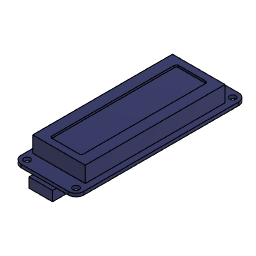
LCD1602 RGB Module v2 (Autodesk Fusion 360 design; units mm, degrees)
Autodesk Fusion 360 part; units mm, degrees
sketch "Skizze1" plane through (0, 0, 0) normal (0, 0, 1) x (1, 0, 0)
  line L0 (4, 0) -> (28, 0)
  line L1 (32, 4) -> (32, 83)
  line L2 (28, 87) -> (4, 87)
  line L3 (0, 83) -> (0, 4)
  circle A0 centre (3.5, 3.5) radius 1.6
  circle A1 centre (28.5, 3.5) radius 1.6
  circle A2 centre (3.5, 83.5) radius 1.6
  circle A3 centre (28.5, 83.5) radius 1.6
  arc A4 (4, 87) -> (0, 83) centre (4, 83) ccw
  arc A5 (32, 83) -> (28, 87) centre (28, 83) ccw
  arc A6 (0, 4) -> (4, 0) centre (4, 4) ccw
  arc A7 (28, 0) -> (32, 4) centre (28, 4) ccw
  point P0 (32, 0)
  point P1 (0, 87)
  dimension "d1" = 32
  dimension "d2" = 87
  dimension "d3" = 3.2
  dimension "d4" = 3.5
  dimension "d5" = 3.5
  dimension "d8" = 25
  dimension "d9" = 80
  dimension "d10" = 4
  constraint horizontal L0
  constraint vertical L1
  constraint horizontal L2
  constraint vertical L3
  constraint coincident P1 L2
  constraint coincident P1 L3
  constraint tangent L2 A4
  constraint tangent L3 A4
  constraint tangent L1 A5
  constraint tangent L2 A5
  constraint equal A4 A5
  constraint coincident origin L0
  constraint coincident origin L3
  constraint tangent L0 A6
  constraint tangent L3 A6
  constraint equal A4 A6
  constraint coincident P0 L0
  constraint coincident P0 L1
  constraint tangent L0 A7
  constraint tangent L1 A7
  constraint equal A4 A7
  measures "d1" distance of origin P0
  measures "d2" distance of origin P1
  measures "d3" diameter of A0
  measures "d4" distance of L0 A0.centre
  measures "d5" distance of L3 A0.centre
  measures "d10" radius of A4
extrude "Extrusion1" add sketch "Skizze1" along normal blind 1.6
sketch "Skizze2" plane through (0, 0, 1.6) normal (0, 0, 1) x (-1, 0, 0)
  circle A0 centre (-28.5, -3.5) radius 1.6
  circle A1 centre (-3.5, -3.5) radius 1.6
  circle A2 centre (-3.5, -83.5) radius 1.6
  circle A3 centre (-28.5, -83.5) radius 1.6
  arc A4 (-28, 0) -> (-32, -4) centre (-28, -4) ccw
  line L0 (-32, -4) -> (-32, -83)
  arc A5 (-32, -83) -> (-28, -87) centre (-28, -83) ccw
  line L1 (-28, -87) -> (-4, -87)
  arc A6 (-4, -87) -> (0, -83) centre (-4, -83) ccw
  line L2 (0, -83) -> (0, -4)
  arc A7 (0, -4) -> (-4, 0) centre (-4, -4) ccw
  line L3 (-4, 0) -> (-28, 0)
  line L4 (-2.08, -7.8) -> (-28.88, -7.8)
  line L5 (-28.88, -7.8) -> (-28.88, -79.1)
  line L6 (-28.88, -79.1) -> (-2.08, -79.1)
  line L7 (-2.08, -79.1) -> (-2.08, -7.8)
  dimension "d13" = 26.8
  dimension "d14" = 71.3
  dimension "d15" = 7.8
  dimension "d16" = 2.08
  constraint horizontal L4
  constraint vertical L5
  constraint horizontal L6
  constraint vertical L7
  measures "d13" distance of L4.start L4.end
  measures "d14" distance of L4.start L6.end
  measures "d15" distance of L3 L4
  measures "d16" distance of L2 L7
extrude "Extrusion2" add sketch "Skizze2" along normal blind 8.1 contours L4 L5 L6 L7
sketch "Skizze3" plane through (0, 0, 9.7) normal (0, 0, 1) x (-1, 0, 0)
  line L0 (-2.08, -79.1) -> (-2.08, -7.8)
  line L1 (-2.08, -7.8) -> (-28.88, -7.8)
  line L2 (-28.88, -7.8) -> (-28.88, -79.1)
  line L3 (-28.88, -79.1) -> (-2.08, -79.1)
  line L4 (-8.48, -11.2) -> (-22.48, -11.2)
  line L5 (-23.48, -12.2) -> (-23.48, -74.7)
  line L6 (-22.48, -75.7) -> (-8.48, -75.7)
  line L7 (-7.48, -74.7) -> (-7.48, -12.2)
  arc A0 (-7.48, -12.2) -> (-8.48, -11.2) centre (-8.48, -12.2) ccw
  arc A1 (-22.48, -11.2) -> (-23.48, -12.2) centre (-22.48, -12.2) ccw
  arc A2 (-8.48, -75.7) -> (-7.48, -74.7) centre (-8.48, -74.7) ccw
  arc A3 (-23.48, -74.7) -> (-22.48, -75.7) centre (-22.48, -74.7) ccw
  point P0 (-7.48, -11.2)
  point P1 (-23.48, -11.2)
  point P2 (-7.48, -75.7)
  dimension "d19" = 16
  dimension "d20" = 64.5
  dimension "d21" = 3.4
  dimension "d22" = 5.4
  dimension "d23" = 1
  constraint horizontal L4
  constraint vertical L5
  constraint horizontal L6
  constraint vertical L7
  constraint coincident P0 L4
  constraint coincident P0 L7
  constraint tangent L4 A0
  constraint tangent L7 A0
  constraint coincident P1 L4
  constraint coincident P1 L5
  constraint tangent L4 A1
  constraint tangent L5 A1
  constraint equal A0 A1
  constraint coincident P2 L6
  constraint coincident P2 L7
  constraint tangent L6 A2
  constraint tangent L7 A2
  constraint equal A0 A2
  constraint tangent L5 A3
  constraint tangent L6 A3
  constraint equal A0 A3
  measures "d19" distance of P0 P1
  measures "d20" distance of P0 P2
  measures "d21" distance of L1 L4
  measures "d22" distance of L0 L7
  measures "d23" radius of A0
extrude "Extrusion3" cut sketch "Skizze3" against normal blind 1 contours L4 L5 L6 L7 A0 A1 A2 A3
sketch "Skizze4" plane through (0, 0, 1.6) normal (0, 0, 1) x (-1, 0, 0)
  line L0 (-2.08, -79.1) -> (-28.88, -79.1)
  line L1 (-28.88, -79.1) -> (-28.88, -7.8)
  line L2 (-28.88, -7.8) -> (-2.08, -7.8)
  line L3 (-2.08, -7.8) -> (-2.08, -79.1)
  circle A0 centre (-28.5, -3.5) radius 1.6
  circle A1 centre (-3.5, -3.5) radius 1.6
  circle A2 centre (-3.5, -83.5) radius 1.6
  circle A3 centre (-28.5, -83.5) radius 1.6
  arc A4 (-28, 0) -> (-32, -4) centre (-28, -4) ccw
  line L4 (-32, -4) -> (-32, -83)
  arc A5 (-32, -83) -> (-28, -87) centre (-28, -83) ccw
  line L5 (-28, -87) -> (-4, -87)
  arc A6 (-4, -87) -> (0, -83) centre (-4, -83) ccw
  line L6 (0, -83) -> (0, -4)
  arc A7 (0, -4) -> (-4, 0) centre (-4, -4) ccw
  line L7 (-4, 0) -> (-28, 0)
  line L8 (-7.48, -79.1) -> (-11.88, -83.5)
  line L9 (-11.88, -83.5) -> (-20.12, -83.5)
  line L10 (-20.12, -83.5) -> (-24.52, -79.1)
  dimension "d26" = 7.48
  dimension "d27" = 7.48
  dimension "d28" = 3.5
  dimension "d29" = 45
  dimension "d30" = 45
  constraint coincident L0 L8.start
  constraint parallel L0 L9
  constraint coincident L0 L10.end
  measures "d26" distance of L6 L8.start
  measures "d27" distance of L4 L10.end
  measures "d28" distance of L5 L9
  measures "d29" angle of L0 L8
  measures "d30" angle of L0 L10
extrude "Extrusion4" add sketch "Skizze4" along normal blind 3 contours L0 L8 L9 L10
sketch "Skizze5" plane through (0, 0, 0) normal (0, 0, -1) x (1, 0, 0)
  circle A0 centre (28.5, -3.5) radius 1.6
  circle A1 centre (3.5, -3.5) radius 1.6
  circle A2 centre (3.5, -83.5) radius 1.6
  circle A3 centre (28.5, -83.5) radius 1.6
  arc A4 (32, -4) -> (28, 0) centre (28, -4) ccw
  line L0 (28, 0) -> (4, 0)
  arc A5 (4, 0) -> (0, -4) centre (4, -4) ccw
  line L1 (0, -4) -> (0, -83)
  arc A6 (0, -83) -> (4, -87) centre (4, -83) ccw
  line L2 (4, -87) -> (28, -87)
  arc A7 (28, -87) -> (32, -83) centre (28, -83) ccw
  line L3 (32, -83) -> (32, -4)
  line L4 (2, -12) -> (5, -12)
  line L5 (5, -12) -> (5, -17)
  line L6 (5, -17) -> (2, -17)
  line L7 (2, -17) -> (2, -12)
  line L8 (30, -12) -> (30, -17)
  line L9 (30, -17) -> (27, -17)
  line L10 (27, -12) -> (30, -12)
  line L11 (27, -17) -> (27, -12)
  line L12 (5, -41) -> (5, -46)
  line L13 (5, -46) -> (2, -46)
  line L14 (2, -41) -> (5, -41)
  line L15 (2, -46) -> (2, -41)
  line L16 (30, -41) -> (30, -46)
  line L17 (30, -46) -> (27, -46)
  line L18 (27, -41) -> (30, -41)
  line L19 (27, -46) -> (27, -41)
  line L20 (5, -70) -> (5, -75)
  line L21 (5, -75) -> (2, -75)
  line L22 (2, -70) -> (5, -70)
  line L23 (2, -75) -> (2, -70)
  line L24 (30, -70) -> (30, -75)
  line L25 (30, -75) -> (27, -75)
  line L26 (27, -70) -> (30, -70)
  line L27 (27, -75) -> (27, -70)
  dimension "d33" = 3
  dimension "d34" = 5
  dimension "d35" = 12
  dimension "d36" = 2
  dimension "d39" = 25
  dimension "d40" = -58
  constraint horizontal L4
  constraint vertical L5
  constraint horizontal L6
  constraint vertical L7
  measures "d33" distance of L4.start L4.end
  measures "d34" distance of L4.start L6.end
  measures "d35" distance of L0 L4
  measures "d36" distance of L1 L7
extrude "Extrusion5" add sketch "Skizze5" along normal blind 2 contours L4 L5 L6 L7 | L8 L9 L10 L11 | L12 L13 L14 L15 | L16 L17 L18 L19 | L20 L21 L22 L23 | L24 L25 L26 L27
sketch "Skizze6" plane through (0, 0, 0) normal (0, 0, -1) x (1, 0, 0)
  line L0 (2, -17) -> (2, -12)
  line L1 (2, -12) -> (5, -12)
  line L2 (5, -12) -> (5, -17)
  line L3 (5, -17) -> (2, -17)
  line L4 (2, -75) -> (2, -70)
  line L5 (2, -70) -> (5, -70)
  line L6 (5, -70) -> (5, -75)
  line L7 (5, -75) -> (2, -75)
  line L8 (2, -46) -> (2, -41)
  line L9 (2, -41) -> (5, -41)
  line L10 (5, -41) -> (5, -46)
  line L11 (5, -46) -> (2, -46)
  line L12 (27, -17) -> (27, -12)
  line L13 (27, -12) -> (30, -12)
  line L14 (30, -12) -> (30, -17)
  line L15 (30, -17) -> (27, -17)
  line L16 (27, -75) -> (27, -70)
  line L17 (27, -70) -> (30, -70)
  line L18 (30, -70) -> (30, -75)
  line L19 (30, -75) -> (27, -75)
  line L20 (27, -46) -> (27, -41)
  line L21 (27, -41) -> (30, -41)
  line L22 (30, -41) -> (30, -46)
  line L23 (30, -46) -> (27, -46)
  circle A0 centre (28.5, -3.5) radius 1.6
  circle A1 centre (3.5, -3.5) radius 1.6
  circle A2 centre (3.5, -83.5) radius 1.6
  circle A3 centre (28.5, -83.5) radius 1.6
  arc A4 (32, -4) -> (28, 0) centre (28, -4) ccw
  line L24 (28, 0) -> (4, 0)
  arc A5 (4, 0) -> (0, -4) centre (4, -4) ccw
  line L25 (0, -4) -> (0, -83)
  arc A6 (0, -83) -> (4, -87) centre (4, -83) ccw
  line L26 (4, -87) -> (28, -87)
  arc A7 (28, -87) -> (32, -83) centre (28, -83) ccw
  line L27 (32, -83) -> (32, -4)
  line L28 (10, 2) -> (22, 2)
  line L29 (22, 2) -> (22, -8)
  line L30 (22, -8) -> (10, -8)
  line L31 (10, -8) -> (10, 2)
  dimension "d43" = 12
  dimension "d44" = 10
  dimension "d45" = 2
  dimension "d46" = 10
  constraint horizontal L28
  constraint vertical L29
  constraint horizontal L30
  constraint vertical L31
  measures "d43" distance of L28.start L28.end
  measures "d44" distance of L28.start L30.end
  measures "d45" distance of L24 L28
  measures "d46" distance of L25 L31
extrude "Extrusion6" add sketch "Skizze6" along normal blind 5 contours L24 L29 L30 L31 | L24 L28 L29 L31
